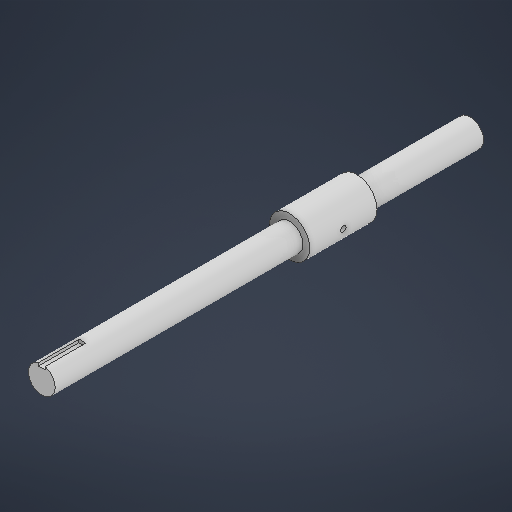
# Autodesk Inventor part: Rough draft shaft
Saved by Autodesk Inventor 2026.3 (Build 303398000, 398)
## iProperties
Created: 2026-07-22
Part Number: Rough draft shaft
Material: Generic
Document SubType Name: Sheet Metal
Designer: matot
Density: 1 g/cm^3
Sheet Metal Rule: Default_mm
Appearance: Default
Author: matot
Autodesk Inventor part; units mm, degrees
ref_plane "YZ Plane" through (0, 0, 0) normal (1, 0, 0) x (0, 1, 0)
ref_plane "XZ Plane" through (0, 0, 0) normal (0, 1, 0) x (-1, 0, 0)
ref_plane "XY Plane" through (0, 0, 0) normal (0, 0, 1) x (1, 0, 0)
sketch "Sketch1" plane through (0, 0, 0) normal (0, 0, 1) x (1, 0, 0)
  circle A0 centre (0, 0) radius 10
  dimension "d0" = 20
  constraints: 1 centre point, 1 coincident
  measures "d0" diameter of A0
extrude "Extrusion1" add sketch "Sketch1" along normal blind 65
sketch "Sketch2" plane through (0, 0, 65) normal (0, 0, 1) x (1, 0, 0)
  circle A0 centre (0, 0) radius 10
  dimension "d3" = 20
  constraints: 1 centre point, 1 coincident
  measures "d3" diameter of A0
extrude "Extrusion2" add sketch "Sketch2" along normal blind 150
sketch "Sketch3" plane through (0, 0, 0) normal (0, 0, -1) x (-1, 0, 0)
  circle A0 centre (0, 0) radius 10
  constraints: 1 centre point, 1 coincident
extrude "Extrusion3" add sketch "Sketch3" along normal blind 100
sketch "Sketch6" plane through (0, 0, -100) normal (0, 0, -1) x (-1, 0, 0)
  circle A0 centre (0, 0) radius 10
  constraints: 1 centre point, 1 coincident
extrude "Extrusion4" cut sketch "Sketch6" against normal blind 54
sketch "Sketch7" plane through (0, 0, 215) normal (0, 0, 1) x (1, 0, 0)
  circle A0 centre (0, 0) radius 10
  constraints: 1 centre point, 1 coincident
extrude "Extrusion5" add sketch "Sketch7" along normal blind 50
ref_plane "Work Plane3" through (0, 0, 81) normal (0, 0, -1) x (-1, 0, 0)
sketch "Sketch9" plane through (0, 0, 81) normal (0, 0, -1) x (-1, 0, 0)
  circle A0 centre (0, 0) radius 15
  dimension "d29" = 30
  constraints: 1 centre point, 1 coincident
  measures "d29" diameter of A0
extrude "Extrusion7" add sketch "Sketch9" along normal blind 50
sketch "Sketch12" plane through (0, 0, -46) normal (0, 0, -1) x (-1, 0, 0)
  circle A0 centre (0, 0) radius 10
  constraints: 1 centre point, 1 coincident
extrude "Extrusion8" add sketch "Sketch12" along normal blind 7.2
sketch "Sketch16" plane through (0, 0, 81) normal (0, 0, -1) x (-1, 0, 0)
  circle A0 centre (0, 0) radius 15 projected
  point P0 (-15, 0)
  constraints: 1 horizontal alignment, 1 other
ref_plane "Work Plane4" through (15, 0, 81) normal (1, 0, 0) x (0, 1, 0)
sketch "Sketch17" plane through (15, 0, 81) normal (1, 0, 0) x (0, 1, 0)
  line L0 (-15, -50) -> (15, -50) projected
  point P0 (0, -81)
  point P1 (0, -25)
  dimension "d67" = 25
  measures "d67" distance from line of point (0, -25) L0
hole "Hole4" at (15, 0, 56) direction (-1, 0, 0) diameter 4 end through all
sketch "Sketch18" plane through (0, 0, 265) normal (0, 0, 1) x (1, 0, 0)
  circle A0 centre (0, 0) radius 10 projected
  line L0 (0, 10) -> (-2.5, 10)
  line L1 (-2.5, 10) -> (-2.5, 7.5)
  line L2 (-2.5, 7.5) -> (0, 7.5)
  line L3 (0, 10) -> (2.5, 10)
  line L4 (2.5, 10) -> (2.5, 7.5)
  line L5 (2.5, 7.5) -> (0, 7.5)
  point P0 (0, 7.5)
  point P1 (2.5, 9.6825)
  point P2 (-2.5, 9.6825)
  dimension "d75" = 5
  dimension "d76" = 2.5
  dimension "d77" = 10
  constraints: 12 end point, 2 horizontal, 2 parallel, 2 perpendicular, 1 point on line, 2 other
  measures "d75" distance of L4.end L1.end
  measures "d76" distance of L4.end L3.end
  measures "d77" distance from line of point (0, 0) L3
extrude "Extrusion12" cut sketch "Sketch18" against normal blind 30 contours L4 L5 L2 L1 A0 picked at (1.3922, 8.2862)
equation "\"d73\" = Thickness"
equation "\"BendRadius\" = Thickness"
equation "\"BendReliefWidth\" = Thickness"
equation "\"BendReliefDepth\" = 0.5 * Thickness"
equation "\"CornerReliefSize\" = 4 * Thickness"
equation "\"MinimumRemnant\" = 2 * Thickness"
equation "\"TransitionRadius\" = BendRadius"
equation "\"JacobiRadiusSize\" = BendRadius"
equation "\"GapSize\" = Thickness"
equation "\"Thickness\" = 0.5"
body "Solid1"
